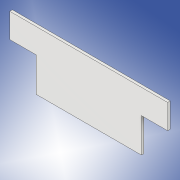
# Autodesk Inventor part: Front Cover
Saved by Autodesk Inventor 2017 SP1 (Build 210196100, 196)
## iProperties
Created: 2017-07-19
Part Number: Front Cover
Material: ABS Plastic
Document SubType Name: Modeling
Designer: zallen
Density: 1.06 g/cm^3
Appearance: CR White
Author: zallen
Autodesk Inventor part; units mm, degrees
ref_plane "YZ Plane" through (0, 0, 0) normal (1, 0, 0) x (0, 1, 0)
ref_plane "XZ Plane" through (0, 0, 0) normal (0, 1, 0) x (-1, 0, 0)
ref_plane "XY Plane" through (0, 0, 0) normal (0, 0, 1) x (1, 0, 0)
sketch "Sketch1" plane through (0, 0, 0) normal (0, 0, 1) x (1, 0, 0)
  line L0 (0, 0) -> (600, 0)
  line L1 (600, 0) -> (600, -93)
  line L2 (600, -93) -> (0, -93)
  line L3 (0, -93) -> (0, 0)
  line L4 (100, -93) -> (500, -93)
  line L5 (500, -93) -> (500, -223)
  line L6 (500, -223) -> (100, -223)
  line L7 (100, -223) -> (100, -93)
  point P0 (300, -93)
  point P1 (300, -223)
  dimension "d0" = 600
  dimension "d1" = 93
  dimension "d2" = 400
  dimension "d6" = 223
  constraints: 16 end point, 4 parallel, 2 horizontal, 2 midpoint, 2 perpendicular, 1 point on line, 1 vertical alignment
  measures "d0" distance of L1.end L2.end
  measures "d1" distance of L0.end L1.end
  measures "d2" distance of L5.end L6.end
  measures "d6" distance between parallel lines of L6 L0
extrude "Extrusion1" add sketch "Sketch1" along normal blind 10
body "Solid1"
